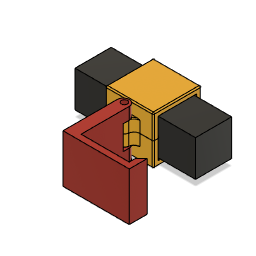
ClampV2 v2 (Autodesk Fusion 360 design; units mm, degrees)
Autodesk Fusion 360 part; units mm, degrees
sketch "Frame" plane through (0, 0, 0) normal (1, 0, 0) x (0, 0, -1)
  line L0 (15, 15) -> (-15, 15)
  line L1 (-15, 15) -> (-15, -15)
  line L2 (-15, -15) -> (15, -15)
  line L3 (15, -15) -> (15, 15)
  dimension "d1" = 30
  dimension "d2" = 30
  constraint horizontal L0
  constraint vertical L1
  constraint horizontal L2
  constraint vertical L3
  measures "d1" distance of L0.start L0.end
  measures "d2" distance of L0.start L2.end
extrude "Extrude1" add sketch "Frame" along normal blind 100 makes body 1
copy_body "Body->Comp1" bodies 1 removing the originals makes body 2 in component "Frame"
sketch "Clamp" plane through (0, 0, 0) normal (1, 0, 0) x (0, 0, -1)
  line L0 (20, 20) -> (0, 20)
  line L1 (0, -20) -> (20, -20)
  line L2 (20, -20) -> (20, 20)
  line L3 (15, 15) -> (0, 15)
  line L4 (0, -15) -> (15, -15)
  line L5 (15, -15) -> (15, 15)
  line L6 (0, 20) -> (0, 15)
  line L7 (0, -15) -> (0, -20)
  constraint horizontal L0
  constraint horizontal L1
  constraint vertical L2
  constraint horizontal L3
  constraint horizontal L4
  constraint vertical L5
  constraint perpendicular L3 L6
extrude "Extrude2" add sketch "Clamp" along normal blind 40 separate body makes body 3
move_body "Move1" bodies 3 to x (1, 0, 0) y (0, 1, 0) z (0, 0, 1) at (30, 0, 0)
move_body "Move2" bodies 3 to x (1, 0, 0) y (0, 0, 1) z (0, -1, 0) at (0, -40, 0)
move_body "Move3" bodies 3 to x (1, 0, 0) y (0, 1, 0) z (0, 0, 1) at (0, 40, 0)
sketch "HolderHoles" plane through (0, 0, 0) normal (0, -1, 0) x (1, 0, 0)
  line L0 (30, -15) -> (30, -20)
  line L1 (30, -20) -> (70, -20)
  line L2 (70, -20) -> (70, -15)
  line L3 (70, -15) -> (30, -15)
  circle A0 centre (50, -23.9496) radius 4
  circle A1 centre (50, -23.9496) radius 2.55
  line L4 (50, -34.7401) -> (50, 30) construction
  line L5 (75, 0) -> (25, 0) construction
  circle A2 centre (50, 23.9496) radius 4
  circle A3 centre (50, 23.9496) radius 2.55
  dimension "d8" = 8
  dimension "d9" = 5.1
  constraint concentric A0 A1
  constraint perpendicular L3 L4
  constraint horizontal L5
  constraint symmetric A0 L5 A2
  constraint symmetric A1 L5 A3
  measures "d8" diameter of A0
  measures "d9" diameter of A1
extrude "Extrude3" add sketch "HolderHoles" against normal blind 10 contours L1 A0 | A2 picked at (49.9365, -20.4689) bodies 3
fillet "Fillet1" radius 5 1 edges at (49.3668, 5, -20) on bodies 3
fillet "Fillet2" radius 5 1 edges at (50.6332, 5, -20) on bodies 3
fillet "Fillet3" radius 5 2 edges at (49.3668, 5, 20) (50.6332, 5, 20) on bodies 3
fillet "Fillet4" radius 1 16 edges at (70, 10, 20) (70, 7.5, 15) (70, 15, 0) (70, 20, 0) (70, 7.5, -15) (70, 10, -20) (50, 20, -20) (50, 20, 20) (50, 0, 15) (50, 0, -15) (30, 20, 0) (30, 10, 20) (30, 10, -20) (30, 7.5, 15) (30, 15, 0) (30, 7.5, -15) on bodies 3
fillet "Fillet5" radius 0.6 8 edges at (44.3843, 10, -21.2638) (50, 10, -27.9496) (55.6157, 10, -21.2638) (47.6226, 10, -24.8717) (55.6157, 10, 21.2638) (50, 10, 27.9496) (44.3843, 10, 21.2638) (47.6226, 10, 23.0275) on bodies 3
copy_body "Body->Comp2" bodies 3 removing the originals makes body 4 in component "Clamp"
sketch "Sketch6" plane through (0, 0, 0) normal (0, 1, 0) x (1, 0, 0)
  line L0 (35, -44.9979) -> (35, -85)
  line L1 (35, -90) -> (25, -90)
  line L2 (25, -90) -> (25, -45)
  line L3 (35, -90) -> (80, -90)
  line L4 (80, -90) -> (80, -85)
  line L5 (75, -85) -> (35, -85)
  line L6 (75, -85) -> (75, -80)
  line L7 (80, -75) -> (80, -85)
  line L8 (75, -80) -> (80, -75)
  circle A0 centre (30, -45) radius 5
  circle A1 centre (30, -44) radius 2.55
  dimension "d30" = 10
  dimension "d32" = 5.1
  dimension "d33" = 1
  constraint vertical L0
  constraint horizontal L1
  constraint vertical L2
  constraint horizontal L3
  constraint vertical L4
  constraint horizontal L5
  constraint vertical L6
  constraint vertical L7
  constraint coincident A0 L0.start
  constraint coincident A0 L2.end
  measures "d30" diameter of A0
  measures "d32" diameter of A1
  measures "d33" distance of A0.centre A1.centre
extrude "Extrude4" add sketch "Sketch6" along normal blind 40 separate body contours A0 | L0 L1 L2 L3 L4 L5 L6 L7 L8 A0 makes body 5
sketch "Sketch7" plane through (25, 0, 0) normal (-1, 0, 0) x (0, 0, 1)
  line L0 (45, 0) -> (90, 0)
  line L1 (90, 0) -> (90, 40)
  line L2 (90, 40) -> (45, 40)
  line L3 (40, 30) -> (50, 30)
  line L4 (50, 30) -> (50, 10)
  line L5 (50, 10) -> (40, 10)
  line L6 (40, 10) -> (40, 30)
  line L7 (45, 40) -> (45, 0)
  dimension "d26" = 20
  dimension "d27" = 10
  constraint horizontal L3
  constraint vertical L4
  constraint horizontal L5
  constraint vertical L6
  measures "d26" distance of L3.start L5.end
  measures "d27" distance of L3.start L3.end
extrude "Extrude5" cut sketch "Sketch7" against normal blind 19 contours L3 L4 L5 L7 | L3 L5 L6 L7 bodies 5
move_body "Move4" bodies 5 to x (1, 0, 0) y (0, 1, 0) z (0, 0, 1) at (20, -20, -20)
component "Frame" placed x (1, 0, 0) y (0, 1, 0) z (0, 0, 1) at (0, 0, 0)
component "Clamp" placed x (1, 0, 0) y (0, 1, 0) z (0, 0, 1) at (0, 0, 0)
component "Clamp" placed x (1, 0, 0) y (0, -1, 0) z (0, 0, -1) at (0, -0.033, 0)
component "Component" placed x (1, 0, 0) y (0, 1, 0) z (0, 0, 1) at (0, 0, 0)
named bodies: "Clamp", "Hook"
